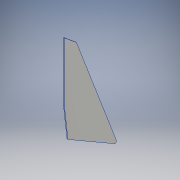
# Autodesk Inventor part: stay_middle
Saved by Autodesk Inventor 2018.1 (Build 221171000, 171)
## iProperties
Created: 2017-10-18
Part Number: stay_middle
Material: アルミニウム 6061
Document SubType Name: Modeling
Designer: kuwano
Density: 2.7 g/cm^3
Appearance: アルミニウム - フラット
Mass: 236.173 g
Surface Area: 610.603 cm^2
Volume: 87.4716 cm^3
Author: kuwano
Autodesk Inventor part; units mm, degrees
ref_plane "YZ Plane" through (0, 0, 0) normal (1, 0, 0) x (0, 1, 0)
ref_plane "XZ Plane" through (0, 0, 0) normal (0, 1, 0) x (-1, 0, 0)
ref_plane "XY Plane" through (0, 0, 0) normal (0, 0, 1) x (1, 0, 0)
sketch "スケッチ1" plane through (0, 0, 0) normal (1, 0, 0) x (0, 1, 0)
  line L0 (-90, 100) -> (-90, -100)
  line L1 (-90, -100) -> (-78.3609, -202.4286)
  line L2 (-78.3609, -202.4286) -> (90, -300)
  line L3 (-126, 0) -> (126, 0) projected
  line L4 (0, -380) -> (0, 180) projected
  line L5 (-90, 100) -> (-49.5962, 66.2658)
  line L6 (-49.5962, 66.2658) -> (90, -300)
  point P0 (-90, 0)
  dimension "d0" = 200
  dimension "d5" = 90
  dimension "d6" = 300
  dimension "d7" = 90
  constraints: 10 end point, 1 midpoint, 1 point on line, 1 vertical
  measures "d0" distance of L0.start L0.end
  measures "d5" distance between parallel lines of L0 L4
  measures "d6" distance from line of L3 L2.end
  measures "d7" distance from line of L4 L2.end
extrude "押し出し1" add sketch "スケッチ1" along normal blind 3 contours L5 L6 L3 L0 | L3 L6 L4 L2 L1 L0 | L6 L2 L4
fillet "フィレット1" radius 5 1 edges at (1.5, 90, -300)
